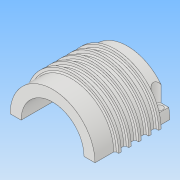
# Autodesk Inventor part: CoreOpposite
Saved by Autodesk Inventor 2017.3 (Build 213256000, 256)
## iProperties
Created: 2019-06-19
Part Number: CoreOpposite
Material: ABS Plastic
Document SubType Name: Modeling
Designer: Derek Wider
Density: 1.06 g/cm^3
Appearance: Smooth - White
Author: Derek Wider
Autodesk Inventor part; units mm, degrees
ref_plane "YZ Plane" through (0, 0, 0) normal (1, 0, 0) x (0, 1, 0)
sketch "Sketch1" plane through (0, 0, 0) normal (0, 0, 1) x (1, 0, 0)
  arc A0 (16.002, 0) -> (-16.002, 0) centre (0, 0) ccw
  arc A1 (21.59, 0) -> (-21.59, 0) centre (0, 0) ccw
  line L0 (-16.002, 0) -> (-21.59, 0)
  line L1 (16.002, 0) -> (21.59, 0)
  dimension "d0" = 43.18
  dimension "d1" = 32.004
  constraints: 4 end point, 4 point on circle, 2 centre point, 2 coincident, 2 point on line, 1 horizontal
  measures "d0" diameter of A1
  measures "d1" diameter of A0
extrude "Extrusion1" add sketch "Sketch1" along normal blind 38.1
ref_plane "Work Plane1" through (0, 0, 27.94) normal (0, 0, 1) x (1, 0, 0)
sketch "Sketch2" plane through (0, 0, 27.94) normal (0, 0, 1) x (1, 0, 0)
  arc A0 (21.59, 0) -> (-21.59, 0) centre (0, 0) ccw projected
  arc A1 (23.495, 0) -> (-23.495, 0) centre (0, 0) ccw
  line L0 (-21.59, 0) -> (-23.495, 0)
  line L1 (16.002, 0) -> (21.59, 0) projected
  line L2 (23.495, 0) -> (21.59, 0)
  dimension "d5" = 1.905
  constraints: 4 end point, 2 point on circle, 1 centre point, 1 collinear
  measures "d5" distance of L0.end L0.start
extrude "Extrusion2" add sketch "Sketch2" against normal blind 1.27
chamfer "Chamfer1" distance 0.635 angle 45 2 edges at (0, 21.59, 27.94) (0, 21.59, 26.67)
pattern_linear "Rectangular Pattern1" count 5 spacing 5.08 along (0, 0, -1) of "Extrusion2", "Chamfer1"
sketch "Sketch3" plane through (16.002, 0, 0) normal (0, -1, 0) x (1, 0, 0)
  line L0 (0, 0) -> (5.588, 0) construction
  line L1 (5.588, 0) -> (5.588, 5.715) construction
  line L2 (6.223, 6.35) -> (5.588, 5.715) construction
  line L3 (7.493, 6.35) -> (6.223, 6.35) construction
  line L4 (7.493, 7.62) -> (7.493, 6.35) construction
  line L5 (7.493, 7.62) -> (6.223, 7.62) construction
  line L6 (5.588, 8.255) -> (6.223, 7.62) construction
  line L7 (5.588, 8.255) -> (5.588, 10.795) construction
  line L8 (6.223, 11.43) -> (5.588, 10.795) construction
  line L9 (7.493, 11.43) -> (6.223, 11.43) construction
  line L10 (7.493, 12.7) -> (7.493, 11.43) construction
  line L11 (7.493, 12.7) -> (6.223, 12.7) construction
  line L12 (5.588, 13.335) -> (6.223, 12.7) construction
  line L13 (5.588, 13.335) -> (5.588, 15.875) construction
  line L14 (6.223, 16.51) -> (5.588, 15.875) construction
  line L15 (7.493, 16.51) -> (6.223, 16.51) construction
  line L16 (7.493, 17.78) -> (7.493, 16.51) construction
  line L17 (7.493, 17.78) -> (6.223, 17.78) construction
  line L18 (5.588, 18.415) -> (6.223, 17.78) construction
  line L19 (5.588, 18.415) -> (5.588, 20.955) construction
  line L20 (6.223, 21.59) -> (5.588, 20.955) construction
  line L21 (7.493, 21.59) -> (6.223, 21.59) construction
  line L22 (7.493, 22.86) -> (7.493, 21.59) construction
  line L23 (7.493, 22.86) -> (6.223, 22.86) construction
  line L24 (5.588, 23.495) -> (6.223, 22.86) construction
  line L25 (5.588, 23.495) -> (5.588, 26.035) construction
  line L26 (6.223, 26.67) -> (5.588, 26.035) construction
  line L27 (7.493, 26.67) -> (6.223, 26.67) construction
  line L28 (7.493, 27.94) -> (7.493, 26.67) construction
  line L29 (7.493, 27.94) -> (6.223, 27.94) construction
  line L30 (5.588, 28.575) -> (6.223, 27.94) construction
  line L31 (5.588, 28.575) -> (5.588, 38.1) construction
  line L32 (0, 38.1) -> (5.588, 38.1) construction
  line L33 (0, 0) -> (0, 38.1) construction
  line L34 (-37.592, 0) -> (-32.004, 0) construction
  line L35 (-32.004, 0) -> (-32.004, 38.1) construction
  line L36 (-37.592, 38.1) -> (-32.004, 38.1) construction
  line L37 (-37.592, 28.575) -> (-37.592, 38.1) construction
  line L38 (-38.227, 27.94) -> (-37.592, 28.575) construction
  line L39 (-38.227, 27.94) -> (-39.497, 27.94) construction
  line L40 (-39.497, 27.94) -> (-39.497, 26.67) construction
  line L41 (-38.227, 26.67) -> (-39.497, 26.67) construction
  line L42 (-37.592, 26.035) -> (-38.227, 26.67) construction
  line L43 (-37.592, 23.495) -> (-37.592, 26.035) construction
  line L44 (-38.227, 22.86) -> (-37.592, 23.495) construction
  line L45 (-38.227, 22.86) -> (-39.497, 22.86) construction
  line L46 (-39.497, 22.86) -> (-39.497, 21.59) construction
  line L47 (-38.227, 21.59) -> (-39.497, 21.59) construction
  line L48 (-37.592, 20.955) -> (-38.227, 21.59) construction
  line L49 (-37.592, 18.415) -> (-37.592, 20.955) construction
  line L50 (-38.227, 17.78) -> (-37.592, 18.415) construction
  line L51 (-38.227, 17.78) -> (-39.497, 17.78) construction
  line L52 (-39.497, 17.78) -> (-39.497, 16.51) construction
  line L53 (-38.227, 16.51) -> (-39.497, 16.51) construction
  line L54 (-37.592, 15.875) -> (-38.227, 16.51) construction
  line L55 (-37.592, 13.335) -> (-37.592, 15.875) construction
  line L56 (-38.227, 12.7) -> (-37.592, 13.335) construction
  line L57 (-38.227, 12.7) -> (-39.497, 12.7) construction
  line L58 (-39.497, 12.7) -> (-39.497, 11.43) construction
  line L59 (-38.227, 11.43) -> (-39.497, 11.43) construction
  line L60 (-37.592, 10.795) -> (-38.227, 11.43) construction
  line L61 (-37.592, 8.255) -> (-37.592, 10.795) construction
  line L62 (-38.227, 7.62) -> (-37.592, 8.255) construction
  line L63 (-38.227, 7.62) -> (-39.497, 7.62) construction
  line L64 (-39.497, 7.62) -> (-39.497, 6.35) construction
  line L65 (-38.227, 6.35) -> (-39.497, 6.35) construction
  line L66 (-37.592, 5.715) -> (-38.227, 6.35) construction
  line L67 (-37.592, 0) -> (-37.592, 5.715) construction
  circle A0 centre (2.794, 2.54) radius 1.778
  circle A1 centre (-34.798, 2.54) radius 1.778
  point P0 (-16.002, 0)
  dimension "d14" = 3.556
  dimension "d15" = 2.54
  dimension "d16" = 3.556
  constraints: 2 centre point, 1 horizontal alignment
  measures "d14" diameter of A0
  measures "d15" distance from line of L0 A0.centre
  measures "d16" diameter of A1
extrude "Extrusion3" cut sketch "Sketch3" against normal through all
ref_plane "Work Plane2" through (16.002, 25.4, 0) normal (0, -1, 0) x (1, 0, 0)
sketch "Sketch4" plane through (16.002, 25.4, 0) normal (0, -1, 0) x (1, 0, 0)
  circle A0 centre (2.794, 2.54) radius 1.778 construction
  circle A1 centre (-34.798, 2.54) radius 1.778 construction
  circle A2 centre (2.794, 2.54) radius 3.048
  circle A3 centre (-34.798, 2.54) radius 3.048
  line L0 (2.794, -0.508) -> (7.3935, -0.1769)
  line L1 (7.3935, -0.1769) -> (6.0075, 2.6942)
  line L2 (6.0075, 2.6942) -> (5.8411, 2.6139)
  line L3 (-34.7976, -0.508) -> (-34.7976, -3.1659)
  line L4 (-34.7976, -3.1659) -> (-38.8338, -2.6207)
  line L5 (-38.8338, -2.6207) -> (-39.8503, 2.0729)
  line L6 (-39.8503, 2.0729) -> (-37.8451, 2.6139)
  point P0 (-16.002, 0)
  dimension "d20" = 6.096
  dimension "d21" = 6.096
  constraints: 14 end point, 4 point on circle, 2 centre point, 2 coincident, 1 perpendicular, 1 vertical
  measures "d20" diameter of A2
  measures "d21" diameter of A3
extrude "Extrusion4" cut sketch "Sketch4" along normal blind 20.32
body "Solid1"
